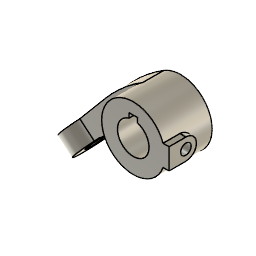
40 (Autodesk Fusion 360 design; units mm, degrees)
Autodesk Fusion 360 part; units mm, degrees
note: some values were not read from the file. Set by a fixed rule: which sketch regions a step uses.
sketch "草图1" plane through (0, 0, 0) normal (0, 1, 0) x (1, 0, 0)
  circle A0 centre (0, 0) radius 30
  arc A1 (-51.6628, 5.5633) -> (-15.811, -25.4954) centre (63.2438, 101.9815) ccw
  arc A2 (-61.753, 45.5913) -> (-8.019, 28.9084) centre (-21.9187, 79.0163) ccw
  line L0 (-51.6628, 5.5633) -> (-136.7415, 106.9562)
  line L1 (-136.7415, 106.9562) -> (-122.9527, 118.5264)
  line L2 (-122.9527, 118.5264) -> (-61.753, 45.5913)
  line L3 (0, -75) -> (0, 85) construction
  line L4 (-4, -14.4568) -> (-4, -19)
  line L5 (-4, -19) -> (4, -19)
  line L6 (4, -19) -> (4, -14.4568)
  arc A3 (4, -14.4568) -> (-4, -14.4568) centre (0, 0) ccw
  line L7 (-150, 0) -> (60, 0) construction
  dimension "d1" = 30
  dimension "d2" = 60
  dimension "d3" = 8
  dimension "d4" = 19
  dimension "d5" = 18
  dimension "d6" = 130
  dimension "d7" = 52
  dimension "d8" = 150
  dimension "d9" = 36
  constraint coincident A0.centre A3.centre
  constraint concentric A0 A3
  constraint coincident A0 A1.end
  constraint tangent A0 A2
  constraint coincident A0 A2.end
  constraint vertical L3
  constraint vertical L4
  constraint perpendicular L4 L5
  constraint perpendicular L5 L6
  constraint symmetric L3 L4 L6
  constraint tangent A1 L0
  constraint tangent A2 L2
  constraint tangent A0 A1
  constraint parallel L0 L2
  constraint perpendicular L1 L2
  constraint horizontal L7
  measures "d1" diameter of A3
  measures "d2" diameter of A0
  measures "d3" distance of L4.end L5.end
  measures "d4" vertical distance of A0.centre L5.end
  measures "d5" distance of L0.end L1.end
  measures "d6" angle of L0 L7
  measures "d7" radius of A2
  measures "d8" radius of A1
  measures "d9" distance of A0.centre L0
extrude "拉伸1" add sketch "草图1" against normal blind 45 contours A0
extrude "拉伸2" add sketch "草图1" against normal blind 20 contours A0 A1 A2 L0 L1 L2
sketch "草图2" plane through (-27.5776, 0, 23.1404) normal (-0.766044, 0, 0.642788) x (0, -1, 0)
  line L0 (0, -37.47) -> (0, -169.829)
  line L1 (0, -169.829) -> (20, -169.829)
  line L2 (20, -169.829) -> (20, -37.47)
  line L3 (20, -37.47) -> (0, -37.47)
  circle A0 centre (10, -90) radius 18
  circle A1 centre (10, -90) radius 8
  line L4 (0, -90) -> (20, -90)
  line L5 (0, -90) -> (-8, -90)
  line L6 (20, -90) -> (28, -90)
  dimension "d14" = 16
  dimension "d15" = 36
  dimension "d16" = 90
  dimension "d17" = 10
  constraint concentric A0 A1
  constraint coincident L0 L4.start
  constraint coincident L2 L4.end
  constraint perpendicular L2 L4
  constraint coincident A0 L5.end
  constraint perpendicular L0 L5
  constraint coincident A0 L6.end
  constraint perpendicular L2 L6
  measures "d14" diameter of A1
  measures "d15" diameter of A0
  measures "d16" vertical distance of origin A0.centre
  measures "d17" horizontal distance of origin A0.centre
extrude "拉伸3" cut sketch "草图2" against normal blind 35 contours L0 L1 L2 A0
extrude "拉伸4" add sketch "草图2" against normal blind 18 contours L0 L2 A0 A1 L4 | L0 A0 L5 | L0 L2 A0 A1 L4 | L0 A0 L5 | L2 A0 L6 | L2 A0 L6
extrude "拉伸5" cut sketch "草图2" against normal blind 25 contours A1 L4 | A1 L4
ref_plane "工作平面1" through (34, 0, 0) normal (1, 0, 0) x (0, 1, 0)
sketch "草图3" plane through (34, 0, 0) normal (1, 0, 0) x (0, 1, 0)
  circle A0 centre (-29, 0) radius 5
  circle A1 centre (-29, 0) radius 10
  line L0 (-29, 10) -> (-45, 10)
  line L1 (-45, 10) -> (-45, -10)
  line L2 (-45, -10) -> (-29, -10)
  line L3 (-100, 0) -> (30, 0) construction
  dimension "d25" = 10
  dimension "d26" = 20
  dimension "d27" = 16
  dimension "d28" = 45
  constraint concentric A0 A1
  constraint coincident A1 L0.start
  constraint horizontal L0
  constraint coincident A1 L2.end
  constraint horizontal L3
  constraint perpendicular L1 L3
  constraint symmetric L0 L2 L3
  constraint tangent A1 L0
  constraint tangent A1 L2
  measures "d25" diameter of A0
  measures "d26" diameter of A1
  measures "d27" distance of A0.centre L1
  measures "d28" distance of origin L1
extrude "拉伸6" add sketch "草图3" against normal blind 10
extrude "拉伸7" cut sketch "草图3" against normal blind 25 contours A0
